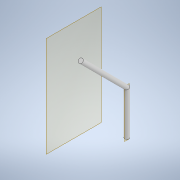
# Autodesk Inventor part: loganFixedPart
Saved by Autodesk Inventor 2022 (Build 260153070, 153G)
## iProperties
Created: 2021-06-06
Part Number: loganFixedPart
Material: Generic
Document SubType Name: Modeling
Designer: robst
Density: 1 g/cm^3
Appearance: Default
Author: robst
Autodesk Inventor part; units mm, degrees
ref_plane "XZ Plane" through (0, 0, 0) normal (0, 1, 0) x (-1, 0, 0)
ref_plane "XY Plane" through (0, 0, 0) normal (0, 0, 1) x (1, 0, 0)
sketch "Sketch1" plane through (0, 0, 0) normal (0, 1, 0) x (-1, 0, 0)
  circle A0 centre (-177.8, 0) radius 12.7
  point P0 (0, 0)
  dimension "d0" = 25.4
  dimension "d1" = 177.8
  constraints: 1 centre point
  measures "d0" diameter of A0
  measures "d1" distance of A0.centre point (0, 0)
sketch "Sketch2" plane through (0, 0, 0) normal (0, 0, 1) x (1, 0, 0)
  line L0 (177.8, 0) -> (177.8, 254)
  point P0 (0, 0)
  dimension "d2" = 177.8
  dimension "d3" = 254
  constraints: 2 end point, 1 vertical
  measures "d2" distance from line of L0 point (0, 0)
  measures "d3" vertical distance of L0.end point (0, 0)
ref_plane "Work Plane1" through (177.8, 0, 0) normal (1, 0, 0) x (0, 1, 0)
sketch "Sketch3" plane through (177.8, 0, 0) normal (1, 0, 0) x (0, 1, 0)
  line L0 (0, 0) -> (254, 0) projected
  line L1 (254, 0) -> (523.4077, 269.4077)
  line L2 (254, 0) -> (635, 0) construction
  dimension "d5" = 381
  dimension "d6" = 45
  constraints: 4 end point, 1 equal length, 1 horizontal
  measures "d5" distance of L0.end L1.end
  measures "d6" angle of L2 L1
sweep "Sweep1" add profiles "Sketch1" path "Sketch3"
body "Solid1"
